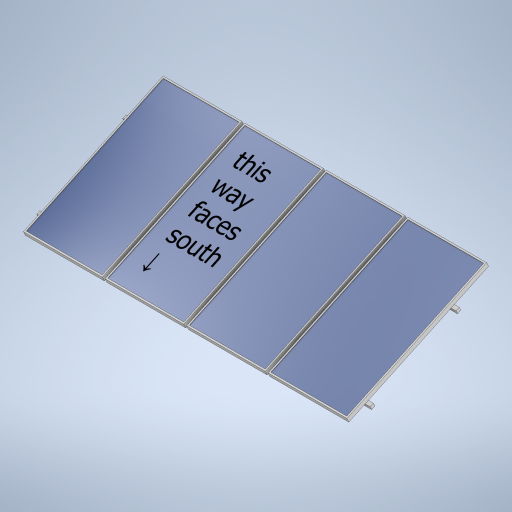
# Autodesk Inventor part: BungaCamp-SolarArray1kW
Saved by Autodesk Inventor 2023 (Build 270158000, 158)
## iProperties
Created: 2024-07-15
Part Number: BungaCamp-SolarArray1kW
Material: Generic
Document SubType Name: Modeling
Designer: incep
Density: 1 g/cm^3
Appearance: Default
Author: incep
Autodesk Inventor part; units mm, degrees
ref_plane "YZ Plane" through (0, 0, 0) normal (1, 0, 0) x (0, 1, 0)
sketch "Sketch1" plane through (0, 0, 0) normal (1, 0, 0) x (0, 1, 0)
  line L0 (162.2592, 725.9074) -> (821.1211, -687.0265)
  line L1 (821.1211, -687.0265) -> (779.4309, -706.4669)
  line L2 (779.4309, -706.4669) -> (120.5691, 706.4669)
  line L3 (120.5691, 706.4669) -> (162.2592, 725.9074)
  line L4 (120.5691, 706.4669) -> (120.5691, -700.6773) construction
  point P0 (0, 0)
  point P1 (450, 0)
  dimension "d0" = 1559
  dimension "d1" = 46
  dimension "d2" = 450
  dimension "d3" = 25
  constraints: 10 end point, 3 perpendicular, 1 horizontal alignment, 1 midpoint, 1 vertical
  measures "d0" distance of L1.end L2.end
  measures "d1" distance of L0.end L1.end
  measures "d2" distance of point (0, 0) point (450, 0)
  measures "d3" angle of L2 L4
extrude "Extrusion1" add sketch "Sketch1" along normal mid plane 798
sketch "Sketch2" plane through (-399, 162.2592, 725.9074) normal (0, 0.9063078, 0.4226183) x (1, 0, 0)
  line L0 (0, 0) -> (798, 0) projected
  line L1 (798, 1559) -> (798, 0) projected
  line L2 (0, 1559) -> (798, 1559) projected
  line L3 (0, 0) -> (0, 1559) projected
  line L4 (783, 15) -> (15, 15)
  line L5 (15, 15) -> (15, 1544)
  line L6 (15, 1544) -> (783, 1544)
  line L7 (783, 1544) -> (783, 15)
  point P0 (399, 589.3218)
  dimension "d6" = 15
  constraints: 8 end point, 3 other
  measures "d6" distance between parallel lines of L0 L4
extrude "Extrusion2" cut sketch "Sketch2" against normal blind 5 contours L4 L5 L6 L7
pattern_linear "Rectangular Pattern1" count 4 spacing 825 along (1, 0, 0)
sketch "Sketch3" plane through (2874, 120.5691, 706.4669) normal (1, 0, 0) x (0, 0.4226183, -0.9063078)
  line L0 (182, 0) -> (218, 0)
  line L1 (218, 0) -> (218, -36)
  line L2 (218, -36) -> (182, -36)
  line L3 (182, -36) -> (182, 0)
  line L4 (1141, 0) -> (1177, 0)
  line L5 (1177, 0) -> (1177, -36)
  line L6 (1177, -36) -> (1141, -36)
  line L7 (1141, -36) -> (1141, 0)
  line L8 (0, 0) -> (1559, 0) projected
  point P0 (589.3218, -407.8385)
  point P1 (200, -36)
  point P2 (1159, -36)
  dimension "d12" = 36
  dimension "d13" = 200
  dimension "d14" = 400
  constraints: 16 end point, 4 parallel, 3 equal length, 2 collinear, 2 horizontal, 2 midpoint, 2 perpendicular
  measures "d12" distance of L1.end L2.end
  measures "d13" horizontal distance of L8.start point (200, -36)
  measures "d14" horizontal distance of L8.end point (1159, -36)
extrude "Extrusion3" add sketch "Sketch3" along normal blind 50
extrude "Extrusion4" add sketch "Sketch3" against normal up to surface (3273 mm away)
sketch "Sketch4" plane through (-399, 0, 0) normal (-1, 0, 0) x (0, 0, 1)
  line L0 (-706.4669, 779.4309) -> (-360.2573, 617.9908) projected
  line L1 (-375.4716, 585.3637) -> (-360.2573, 617.9908) projected
  line L2 (-342.8445, 570.1494) -> (-375.4716, 585.3637) projected
  line L3 (-327.6303, 602.7765) -> (-342.8445, 570.1494) projected
  line L4 (-327.6303, 602.7765) -> (508.8918, 212.6998) projected
  line L5 (493.6776, 180.0728) -> (508.8918, 212.6998) projected
  line L6 (526.3046, 164.8585) -> (493.6776, 180.0728) projected
  line L7 (541.5189, 197.4856) -> (526.3046, 164.8585) projected
  line L8 (541.5189, 197.4856) -> (706.4669, 120.5691) projected
  line L9 (706.4669, 120.5691) -> (725.9074, 162.2592) projected
  line L10 (725.9074, 162.2592) -> (-687.0265, 821.1211) projected
  line L11 (-687.0265, 821.1211) -> (-706.4669, 779.4309) projected
  line L12 (-706.4669, 779.4309) -> (-360.2573, 617.9908) projected
  line L13 (-327.6303, 602.7765) -> (-360.2573, 617.9908) projected
  line L14 (-360.2573, 617.9908) -> (-327.6303, 602.7765)
  line L15 (541.5189, 197.4856) -> (508.8918, 212.6998) projected
  line L16 (706.4669, 120.5691) -> (541.5189, 197.4856) projected
  line L17 (508.8918, 212.6998) -> (541.5189, 197.4856)
  point P0 (0, 0)
  constraints: 4 end point, 1 collinear, 1 perpendicular
extrude "Extrusion5" add sketch "Sketch4" along normal blind 50 contours L13 L3 L2 L1 | L15 L7 L6 L5
ref_plane "Work Plane1" through (1874, 162.2592, 725.9074) normal (1, 0, 0) x (0, 0.4226183, -0.9063078)
sketch "Sketch5" plane through (1874, 162.2592, 725.9074) normal (1, 0, 0) x (0, 0.4226183, -0.9063078)
  line L0 (182, -82) -> (112.3278, -231.4125)
  line L1 (112.3278, -231.4125) -> (141.898, -245.2013)
  line L2 (218, -82) -> (218, -46) projected
  line L3 (141.898, -245.2013) -> (218, -82)
  line L4 (0, -46) -> (1812.6156, -891.2365) construction
  line L5 (0, -46) -> (182, -46) construction
  line L6 (-316.986, -31.2202) -> (1495.6296, -876.4568) construction
  line L7 (81.7975, -217.176) -> (172.4283, -259.4379)
  line L8 (172.4283, -259.4379) -> (181.7544, -239.4379)
  line L9 (181.7544, -239.4379) -> (91.1236, -197.176)
  line L10 (91.1236, -197.176) -> (81.7975, -217.176)
  line L11 (1141, -82) -> (900.0444, -598.7309)
  line L12 (900.0444, -598.7309) -> (929.6146, -612.5197)
  line L13 (929.6146, -612.5197) -> (1177, -82)
  line L14 (959.3088, -628.4636) -> (870.3502, -582.7869)
  line L15 (870.3502, -582.7869) -> (880.43, -563.1559)
  line L16 (880.43, -563.1559) -> (969.3886, -608.8326)
  line L17 (969.3886, -608.8326) -> (959.3088, -628.4636)
  line L18 (218, -82) -> (218, -46) projected
  line L19 (218, -46) -> (182, -46) projected
  line L20 (182, -46) -> (182, -82) projected
  line L21 (182, -82) -> (218, -82) projected
  line L22 (1177, -82) -> (1177, -46) projected
  line L23 (1177, -46) -> (1141, -46) projected
  line L24 (1141, -46) -> (1141, -82) projected
  line L25 (1141, -82) -> (1177, -82) projected
  point P0 (589.3218, -453.8385)
  point P1 (589.3218, -453.8385)
  point P2 (127.1129, -238.3069)
  point P3 (127.1129, -238.3069)
  point P4 (914.8295, -605.6253)
  point P5 (589.3218, -453.8385)
  point P6 (1141, -82)
  point P7 (909.6396, -578.1539)
  point P8 (938.6852, -593.0677)
  point P9 (218, -82)
  point P10 (182, -82)
  point P11 (121.6539, -211.4125)
  point P12 (151.2241, -225.2013)
  point P13 (112.3278, -231.4125)
  point P14 (141.898, -245.2013)
  dimension "d22" = 25
  dimension "d23" = 2000
  dimension "d24" = 100
  dimension "d25" = 20
  constraints: 32 end point, 9 perpendicular, 5 midpoint, 4 parallel, 4 point on line, 3 equal length, 2 coincident
  measures "d22" angle of L5 L4
  measures "d23" distance of L6.start L6.end
  measures "d24" distance of L8.end L9.end
  measures "d25" vertical distance of L7.end L8.end
extrude "Extrusion6" add sketch "Sketch5" along normal mid plane 36 contours L21 L3 L9 L0 | L25 L13 L16 L11
extrude "Extrusion7" add sketch "Sketch5" along normal mid plane 100 contours L9 L3 L1 L0 | L0 L7 L10 L9 | L9 L8 L7 L3 | L16 L13 L12 L14 L11 | L11 L14 L15 L16 | L16 L17 L14 L12 L13
ref_plane "Work Plane2" through (1237.5, 162.2592, 725.9074) normal (1, 0, 0) x (0, 0.4226183, -0.9063078)
mirror "Mirror1" about plane through (1237.5, 162.2592, 725.9074) normal (1, 0, 0) of "Extrusion7", "Extrusion6"
sketch "Sketch6" plane through (426, 162.2592, 725.9074) normal (0, 0.9063078, 0.4226183) x (1, 0, 0)
  line L0 (158.5781, 1382.168) -> (428.0271, 1382.168) construction
  line L1 (428.0271, 1382.168) -> (428.0271, 1355.4743) construction
  line L2 (428.0271, 1355.4743) -> (158.5781, 1355.4743) construction
  line L3 (158.5781, 1355.4743) -> (158.5781, 1382.168) construction
  constraints: 2 other
body "Solid1"
